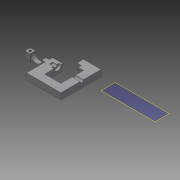
# Autodesk Inventor part: gear frame 1
Saved by Autodesk Inventor 2016 (Build 200138000, 138)
## iProperties
Created: 2017-06-15
Part Number: gear frame 1
Material: Generic
Document SubType Name: Modeling
Designer: RMcComber
Density: 1 g/cm^3
Appearance: Default
d0: 12.700 mm
d1: 2.000 mm
d2: 1.000 mm
d3: 20.000 mm
d4: 16.000 mm
d5: 10.000 mm
d6: 40.000 mm
d7: 25.000 mm
d8: 50.000 mm
d9: 20.000 mm
d10: 20.000 mm
d11: 15.000 mm
d12: 14.000 mm
d13: 25.000 mm
d14: 20.000 mm
d15: 0.00 deg
d16: 34.925 mm
d18: 0.00 deg
d19: 16.000 mm
d20: 16.000 mm
d22: 0.00 deg
d23: 8.000 mm
d25: 0.00 deg
d26: 10.000 mm
d27: 95.000 mm
d28: 0.00 deg
d29: 22.000 mm
d30: 7.000 mm
d31: 0.00 deg
d32: 22.000 mm
d33: 15.000 mm
d34: 0.00 deg
d35: 16.000 mm
d36: 16.000 mm
d38: 0.00 deg
d39: 8.000 mm
d41: 0.00 deg
d42: 8.000 mm
d43: 8.000 mm
d46: 8.000 mm
d47: 25.000 mm
d48: 8.000 mm
d49: 8.000 mm
d50: 12.000 mm
d51: 15.000 mm
d52: 15.000 mm
d53: 8.000 mm
d54: 40.000 mm
d55: 10.000 mm
d57: 0.00 deg
d58: 5.000 mm
d61: 10.000 mm
d64: 5.000 mm
d67: 5.000 mm
d70: 10.000 mm
d73: 10.000 mm
d76: 10.000 mm
d79: 5.000 mm
Author: RMcComber
Autodesk Inventor part; units mm, degrees
ref_plane "YZ Plane" through (0, 0, 0) normal (1, 0, 0) x (0, 1, 0)
ref_plane "XZ Plane" through (0, 0, 0) normal (0, 1, 0) x (-1, 0, 0)
ref_plane "XY Plane" through (0, 0, 0) normal (0, 0, 1) x (1, 0, 0)
ref_plane "Work Plane1" through (-191.4749, 128.3402, -15) normal (0, 0, -1) x (-1, 0, 0)
sketch "Sketch1" plane through (-191.4749, 128.3402, -15) normal (0, 0, -1) x (-1, 0, 0)
  line L0 (190.8, 9) -> (190.8, -9) construction
  line L1 (221.5, 38.1385) -> (221.5, 59.5385) construction
  line L2 (228.2, 37.8385) -> (228.2, 59.8385) construction
  line L3 (292.4096, 87.8385) -> (292.4096, -112.1615) construction
  line L4 (308.2846, 87.8385) -> (308.2846, -112.1615) construction
  line L5 (240.5, -40) -> (240.5, 20.35)
  line L6 (240.5, 20.35) -> (277.4096, 20.35)
  line L7 (277.4096, 20.35) -> (277.4096, 6.35)
  line L8 (277.4096, 6.35) -> (328.2846, 6.35)
  line L9 (328.2846, 6.35) -> (328.2846, -6.35)
  line L10 (328.2846, -6.35) -> (272.4096, -6.35)
  line L11 (272.4096, -6.35) -> (272.4096, -65)
  line L12 (272.4096, -65) -> (165.5, -65)
  line L13 (165.5, -65) -> (165.5, 60.1385)
  line L14 (165.5, 60.1385) -> (220.5, 60.1385)
  line L15 (220.5, 60.1385) -> (220.5, 40.1385)
  line L16 (220.5, 40.1385) -> (190.5, 40.1385)
  line L17 (190.5, 40.1385) -> (206.5, 40.1385)
  line L18 (206.5, 40.1385) -> (206.5, 30.1385)
  line L19 (206.5, 30.1385) -> (190.5, 30.1385)
  line L20 (190.5, 30.1385) -> (190.5, 40.1385)
  line L21 (190.5, 30.1385) -> (190.5, -40)
  line L22 (190.5, -40) -> (240.5, -40)
  line L23 (190.5, -8.7) -> (190.5, 8.7) construction
  point P0 (-191.4749, -128.3402)
  point P1 (328.2846, 0)
  point P2 (190.8, 0)
  point P3 (190.5, 0)
  dimension "d0" = 12.7
  dimension "d1" = 2
  dimension "d2" = 1
  dimension "d3" = 20
  dimension "d4" = 16
  dimension "d5" = 10
  dimension "d6" = 40
  dimension "d7" = 25
  dimension "d8" = 50
  dimension "d9" = 20
  dimension "d10" = 20
  dimension "d11" = 15
  dimension "d12" = 14
  dimension "d13" = 25
  constraints: 40 end point, 8 parallel, 8 perpendicular, 3 midpoint, 2 vertical, 1 collinear, 1 horizontal, 1 horizontal alignment, 1 point on line, 4 other
  measures "d0" distance of L8.end L9.end
  measures "d1" distance from line of L1.start L16
  measures "d2" distance between parallel lines of L1 L15
  measures "d3" distance between parallel lines of L16 L14
  measures "d4" distance of L18.end L19.end
  measures "d5" distance of L17.end L18.end
  measures "d6" distance from line of point (190.5, 0) L22
  measures "d7" distance between parallel lines of L21 L13
  measures "d8" distance of L21.end L5.start
  measures "d9" distance between parallel lines of L9 L4
  measures "d10" distance between parallel lines of L3 L11
  measures "d11" distance between parallel lines of L3 L7
  measures "d12" distance between parallel lines of L8 L6
  measures "d13" distance between parallel lines of L12 L22
extrude "Extrusion1" add sketch "Sketch1" along normal blind 20
sketch "Sketch2" plane through (-519.7595, 121.9902, -15) normal (0, -1, 0) x (1, 0, 0)
  circle A0 centre (27.9375, 0) radius 30 construction
  circle A1 centre (27.9375, 0) radius 17.4625
  point P0 (519.7595, 15)
  dimension "d16" = 34.925
  constraints: 1 centre point, 1 coincident
  measures "d16" diameter of A1
extrude "Extrusion2" cut sketch "Sketch2" against normal through all
sketch "Sketch3" plane through (-191.4749, 128.3402, -15) normal (0, 0, 1) x (1, 0, 0)
  line L0 (-317.8096, -6.35) -> (-317.8096, 6.35) projected
  line L1 (-333.8096, 8) -> (-317.8096, 8)
  line L2 (-317.8096, 8) -> (-317.8096, -8)
  line L3 (-317.8096, -8) -> (-333.8096, -8)
  line L4 (-333.8096, -8) -> (-333.8096, 8)
  point P0 (191.4749, -128.3402)
  point P1 (-317.8096, 0)
  dimension "d19" = 16
  dimension "d20" = 16
  constraints: 8 end point, 2 midpoint, 2 parallel, 1 horizontal, 1 perpendicular
  measures "d19" distance of L3.end L1.start
  measures "d20" distance of L1.start L1.end
extrude "Extrusion3" add sketch "Sketch3" against normal up to surface (20 mm away)
sketch "Sketch4" plane through (-191.4749, 128.3402, -35) normal (0, 0, -1) x (-1, 0, 0)
  line L0 (317.8096, -8) -> (333.8096, -8) projected
  line L1 (333.8096, 8) -> (317.8096, 8) projected
  line L2 (325.8096, 8) -> (325.8096, -8)
  circle A0 centre (325.8096, 0) radius 4
  point P0 (-191.4749, -128.3402)
  dimension "d23" = 8
  constraints: 3 midpoint, 2 end point, 1 centre point
  measures "d23" diameter of A0
extrude "Extrusion4" cut sketch "Sketch4" against normal through all
sketch "Sketch5" plane through (-356.9749, 63.3402, -15) normal (1, 0, 0) x (0, 0, -1)
  arc A0 (1.3364, 96.1329) -> (-1.3364, 96.1329) centre (0, 65) ccw construction
  arc A1 (-1.3364, 96.1329) -> (-7.1127, 95.3389) centre (0, 65) ccw construction
  arc A2 (-7.1127, 95.3389) -> (-9.6864, 94.6178) centre (0, 65) ccw construction
  arc A3 (-9.6864, 94.6178) -> (-15.0343, 92.2949) centre (0, 65) ccw construction
  arc A4 (-15.0343, 92.2949) -> (-17.318, 90.9062) centre (0, 65) ccw construction
  arc A5 (-17.318, 90.9062) -> (-21.8409, 87.2265) centre (0, 65) ccw construction
  arc A6 (-21.8409, 87.2265) -> (-23.6652, 85.2731) centre (0, 65) ccw construction
  arc A7 (-23.6652, 85.2731) -> (-27.0276, 80.5097) centre (0, 65) ccw construction
  arc A8 (-27.0276, 80.5097) -> (-28.2572, 78.1366) centre (0, 65) ccw construction
  arc A9 (-28.2572, 78.1366) -> (-30.2098, 72.6426) centre (0, 65) ccw construction
  arc A10 (-30.2098, 72.6426) -> (-30.7536, 70.0257) centre (0, 65) ccw construction
  arc A11 (-30.7536, 70.0257) -> (-31.1515, 64.2087) centre (0, 65) ccw construction
  arc A12 (-31.1515, 64.2087) -> (-30.9691, 61.5421) centre (0, 65) ccw construction
  arc A13 (-30.9691, 61.5421) -> (-29.7828, 55.8335) centre (0, 65) ccw construction
  arc A14 (-29.7828, 55.8335) -> (-28.8878, 53.315) centre (0, 65) ccw construction
  arc A15 (-28.8878, 53.315) -> (-26.2053, 48.1381) centre (0, 65) ccw construction
  arc A16 (-26.2053, 48.1381) -> (-24.6639, 45.9545) centre (0, 65) ccw construction
  arc A17 (-24.6639, 45.9545) -> (-20.6842, 41.6933) centre (0, 65) ccw construction
  arc A18 (-20.6842, 41.6933) -> (-18.6109, 40.0065) centre (0, 65) ccw construction
  arc A19 (-18.6109, 40.0065) -> (-13.6291, 36.977) centre (0, 65) ccw construction
  arc A20 (-13.6291, 36.977) -> (-11.1776, 35.9122) centre (0, 65) ccw construction
  arc A21 (-11.1776, 35.9122) -> (-5.5632, 34.3391) centre (0, 65) ccw construction
  arc A22 (-5.5632, 34.3391) -> (-2.9153, 33.9751) centre (0, 65) ccw construction
  arc A23 (-2.9153, 33.9751) -> (2.9153, 33.9751) centre (0, 65) ccw construction
  arc A24 (2.9153, 33.9751) -> (5.5632, 34.3391) centre (0, 65) ccw construction
  arc A25 (5.5632, 34.3391) -> (11.1776, 35.9122) centre (0, 65) ccw construction
  arc A26 (11.1776, 35.9122) -> (13.6291, 36.977) centre (0, 65) ccw construction
  arc A27 (13.6291, 36.977) -> (18.6109, 40.0065) centre (0, 65) ccw construction
  arc A28 (18.6109, 40.0065) -> (20.6842, 41.6933) centre (0, 65) ccw construction
  arc A29 (20.6842, 41.6933) -> (24.6639, 45.9545) centre (0, 65) ccw construction
  arc A30 (24.6639, 45.9545) -> (26.2053, 48.1381) centre (0, 65) ccw construction
  arc A31 (26.2053, 48.1381) -> (28.8878, 53.315) centre (0, 65) ccw construction
  arc A32 (28.8878, 53.315) -> (29.7828, 55.8335) centre (0, 65) ccw construction
  arc A33 (29.7828, 55.8335) -> (30.9691, 61.5421) centre (0, 65) ccw construction
  arc A34 (30.9691, 61.5421) -> (31.1515, 64.2087) centre (0, 65) ccw construction
  arc A35 (31.1515, 64.2087) -> (30.7536, 70.0257) centre (0, 65) ccw construction
  arc A36 (30.7536, 70.0257) -> (30.2098, 72.6426) centre (0, 65) ccw construction
  arc A37 (30.2098, 72.6426) -> (28.2572, 78.1366) centre (0, 65) ccw construction
  arc A38 (28.2572, 78.1366) -> (27.0276, 80.5097) centre (0, 65) ccw construction
  arc A39 (27.0276, 80.5097) -> (23.6652, 85.2731) centre (0, 65) ccw construction
  arc A40 (23.6652, 85.2731) -> (21.8409, 87.2265) centre (0, 65) ccw construction
  arc A41 (21.8409, 87.2265) -> (17.318, 90.9062) centre (0, 65) ccw construction
  arc A42 (17.318, 90.9062) -> (15.0343, 92.2949) centre (0, 65) ccw construction
  arc A43 (15.0343, 92.2949) -> (9.6864, 94.6178) centre (0, 65) ccw construction
  arc A44 (9.6864, 94.6178) -> (7.1127, 95.3389) centre (0, 65) ccw construction
  arc A45 (7.1127, 95.3389) -> (1.3364, 96.1329) centre (0, 65) ccw construction
  circle A46 centre (-10, 65) radius 3 construction
  arc A47 (7, 65) -> (-7, 65) centre (0, 65) ccw construction
  circle A48 centre (10, 65) radius 3 construction
  arc A49 (-7, 65) -> (7, 65) centre (0, 65) ccw construction
  circle A50 centre (0, 65) radius 5
  point P0 (-15, -63.3402)
  dimension "d26" = 10
  constraints: 1 centre point, 1 coincident, 1 horizontal alignment
  measures "d26" diameter of A50
extrude "Extrusion5" cut sketch "Sketch5" against normal blind 95
sketch "Sketch6" plane through (-431.9749, 88.3402, -35) normal (1, 0, 0) x (0, 0, -1)
  arc A0 (-20, 35) -> (-20, 45) centre (-20, 40) ccw projected
  circle A1 centre (-20, 40) radius 11
  point P0 (-35, -88.3402)
  dimension "d29" = 22
  constraints: 1 centre point, 1 coincident
  measures "d29" diameter of A1
extrude "Extrusion6" cut sketch "Sketch6" against normal blind 7
sketch "Sketch7" plane through (-356.9749, 63.3402, -35) normal (1, 0, 0) x (0, 0, -1)
  arc A0 (-20, 60) -> (-20, 70) centre (-20, 65) ccw projected
  circle A1 centre (-20, 65) radius 11
  point P0 (-35, -63.3402)
  dimension "d32" = 22
  constraints: 1 centre point, 1 coincident
  measures "d32" diameter of A1
extrude "Extrusion7" cut sketch "Sketch7" against normal blind 15
sketch "Sketch8" plane through (-191.4749, 128.3402, -35) normal (0, 0, -1) x (-1, 0, 0)
  line L0 (220.5, 60.1385) -> (204.5, 60.1385)
  line L1 (204.5, 60.1385) -> (204.5, 76.1385)
  line L2 (204.5, 76.1385) -> (220.5, 76.1385)
  line L3 (220.5, 76.1385) -> (220.5, 60.1385)
  point P0 (-191.4749, -128.3402)
  dimension "d35" = 16
  dimension "d36" = 16
  constraints: 8 end point, 2 parallel, 1 horizontal, 1 perpendicular
  measures "d35" distance of L0.end L1.end
  measures "d36" distance of L1.end L2.end
extrude "Extrusion8" add sketch "Sketch8" against normal up to surface (20 mm away)
sketch "Sketch9" plane through (-356.9749, 63.3402, -35) normal (1, 0, 0) x (0, 0, -1)
  circle A0 centre (-20, 113.8385) radius 10.7 projected
  circle A1 centre (-20, 113.8385) radius 10.7 projected
  circle A2 centre (-20, 113.8385) radius 4
  point P0 (-35, -63.3402)
  dimension "d39" = 8
  constraints: 1 centre point, 1 coincident
  measures "d39" diameter of A2
extrude "Extrusion9" cut sketch "Sketch9" against normal through all contours A2
sketch "Sketch10" plane through (-191.4749, 128.3402, -35) normal (0, 0, -1) x (-1, 0, 0)
  line L0 (277.4096, 6.35) -> (277.4096, 20.35) projected
  line L1 (190.5, 30.1385) -> (206.5, 30.1385) projected
  line L2 (220.5, 40.1385) -> (220.5, 76.1385) projected
  line L3 (204.5, 76.1385) -> (204.5, 60.1385) projected
  line L4 (165.5, 60.1385) -> (165.5, -65) projected
  line L5 (165.5, -65) -> (272.4096, -65) projected
  line L6 (204.5, 68.1385) -> (220.5, 68.1385) construction
  line L7 (198.5, 30.1385) -> (198.5, 40.1385) construction
  line L8 (198.5, 40.1385) -> (206.5, 40.1385) construction
  circle A0 centre (198.5, 40.1385) radius 4
  circle A1 centre (212.5, 68.1385) radius 4
  line L9 (247.5, 11) -> (240.5, 11) construction
  line L10 (240.5, -11) -> (247.5, -11) construction
  line L11 (247.5, 11) -> (247.5, -11) construction
  line L12 (282.8846, 6.35) -> (282.8846, -6.35) construction
  line L13 (247.5, 0) -> (255.5, 0) construction
  line L14 (255.5, 12.5) -> (255.5, -12.5) construction
  line L15 (260.5, 5) -> (247.5, 5) construction
  line L16 (247.5, -5) -> (260.5, -5) construction
  circle A2 centre (255.5, 12.5) radius 4
  circle A3 centre (255.5, -12.5) radius 4
  line L17 (180.5, -53) -> (257.4096, -53) construction
  circle A4 centre (180.5, -53) radius 4
  circle A5 centre (257.4096, -53) radius 4
  line L18 (272.4096, -65) -> (272.4096, -6.35) projected
  line L19 (180.5, -5) -> (190.5, -5) construction
  line L20 (190.5, 5) -> (180.5, 5) construction
  line L21 (180.5, 11) -> (165.5, 11) construction
  line L22 (165.5, -11) -> (180.5, -11) construction
  line L23 (175.5, 20) -> (175.5, -20) construction
  circle A6 centre (175.5, 20) radius 4
  circle A7 centre (175.5, -20) radius 4
  line L24 (165.5, -11) -> (165.5, 11) projected
  point P0 (-191.4749, -128.3402)
  point P1 (175.5, 0)
  point P2 (165.5, 0)
  dimension "d42" = 8
  dimension "d43" = 8
  dimension "d46" = 8
  dimension "d47" = 25
  dimension "d48" = 8
  dimension "d49" = 8
  dimension "d50" = 12
  dimension "d51" = 15
  dimension "d52" = 15
  dimension "d53" = 8
  dimension "d54" = 40
  dimension "d55" = 10
  constraints: 16 end point, 8 centre point, 7 coincident, 7 midpoint, 7 perpendicular, 3 equal radius, 2 parallel, 1 horizontal alignment, 1 point on line
  measures "d42" diameter of A0
  measures "d43" diameter of A1
  measures "d46" diameter of A2
  measures "d47" distance of L14.start L14.end
  measures "d48" distance of L13.start L13.end
  measures "d49" diameter of A4
  measures "d50" distance between parallel lines of L5 L17
  measures "d51" distance from line of L18 L17.end
  measures "d52" distance from line of L4 L17.start
  measures "d53" diameter of A6
  measures "d54" distance of L23.start L23.end
  measures "d55" distance between parallel lines of L24 L23
extrude "Extrusion10" cut sketch "Sketch10" against normal through all
chamfer "Chamfer1" distance 5 angle 45 2 edges at (-397.9749, 168.4787, -25) (-397.9749, 158.4787, -25)
chamfer "Chamfer2" distance 10 angle 45 2 edges at (-395.9749, 188.4787, -25) (-381.9749, 158.4787, -25)
chamfer "Chamfer3" distance 5 angle 45 3 edges at (-395.9749, 204.4787, -25) (-411.9749, 204.4787, -25) (-411.9749, 168.4787, -25)
chamfer "Chamfer4" distance 5 angle 45 1 edges at (-356.9749, 188.4787, -25)
chamfer "Chamfer5" distance 10 angle 45 2 edges at (-356.9749, 63.3402, -25) (-463.8845, 63.3402, -25)
chamfer "Chamfer6" distance 10 angle 45 2 edges at (-381.9749, 88.3402, -25) (-431.9749, 88.3402, -25)
chamfer "Chamfer7" distance 10 angle 45 2 edges at (-468.8845, 148.6902, -25) (-463.8845, 121.9902, -25)
chamfer "Chamfer8" distance 5 angle 45 1 edges at (-431.9749, 148.6902, -25)
body "Solid1"
